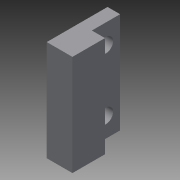
# Autodesk Inventor part: reed_switch
Saved by Autodesk Inventor 2015 SP1 (Build 190203100, 203)
## iProperties
Created: 2016-10-26
Part Number: reed_switch
Material: Generic
Document SubType Name: Modeling
Designer: lustinga
Density: 1 g/cm^3
Appearance: Default
Author: lustinga
Autodesk Inventor part; units mm, degrees
ref_plane "YZ Plane" through (0, 0, 0) normal (1, 0, 0) x (0, 1, 0)
ref_plane "XZ Plane" through (0, 0, 0) normal (0, 1, 0) x (-1, 0, 0)
ref_plane "XY Plane" through (0, 0, 0) normal (0, 0, 1) x (1, 0, 0)
sketch "Sketch1" plane through (0, 0, 0) normal (1, 0, 0) x (0, 1, 0)
  line L0 (9.6754, 10.4121) -> (-4.2246, 10.4121)
  line L1 (-4.2246, 10.4121) -> (-4.2246, -12.5879)
  line L2 (-4.2246, -12.5879) -> (9.6754, -12.5879)
  line L3 (9.6754, -12.5879) -> (9.6754, 10.4121)
  line L4 (9.6754, -1.0879) -> (8.0754, -1.0879) construction
  line L5 (8.0754, -1.0879) -> (8.0754, -8.0879) construction
  line L6 (8.0754, -8.0879) -> (8.0754, 5.9121) construction
  line L7 (8.0754, 5.9121) -> (6.4254, 5.9121) construction
  circle A0 centre (6.4254, 5.9121) radius 1.65
  circle A1 centre (6.4254, -8.0879) radius 1.65
  point P0 (0, 0)
  dimension "d0" = 13.9
  dimension "d1" = 23
  dimension "d7" = 1.6
  dimension "d8" = 7
  dimension "d9" = 90
  dimension "d10" = 14
  dimension "d11" = 1.65
  dimension "d12" = 3.3
  dimension "d13" = 3.3
  constraints: 16 end point, 3 horizontal, 2 centre point, 2 parallel, 2 perpendicular, 1 coincident, 1 midpoint, 1 point on line
  measures "d0" distance of L2.end L1.end
  measures "d1" distance of L1.end L0.end
  measures "d7" distance of L4.start L4.end
  measures "d8" distance of L4.end L5.end
  measures "d9" angle of L5 L4
  measures "d10" distance of L5.end L6.end
  measures "d11" distance of L6.end L7.end
  measures "d12" diameter of A0
  measures "d13" diameter of A1
extrude "Extrusion1" add sketch "Sketch1" along normal blind 2.87
sketch "Sketch2" plane through (2.87, 0, 0) normal (1, 0, 0) x (0, 0, -1)
  line L0 (12.5879, -4.2246) -> (12.5879, 9.6754) projected
  line L1 (-10.4121, -4.2246) -> (12.5879, -4.2246)
  line L2 (12.5879, -4.2246) -> (12.5879, 3.2154)
  line L3 (12.5879, 3.2154) -> (-10.4121, 3.2154)
  line L4 (-10.4121, 3.2154) -> (-10.4121, -4.2246)
  point P0 (0, 0)
  dimension "d4" = 7.44
  constraints: 8 end point, 2 parallel, 1 horizontal, 1 perpendicular, 1 point on line
  measures "d4" distance of L2.end L1.end
extrude "Extrusion2" add sketch "Sketch2" along normal blind 3
body "Solid1"
